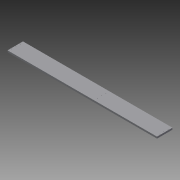
# Autodesk Inventor part: licht_200_back1
Saved by Autodesk Inventor 2015 (Build 190159000, 159)
## iProperties
Created: 2018-01-11
Part Number: licht_200_back1
Material: Generisch
Document SubType Name: Modeling
Designer: schueler
Density: 1 g/cm^3
Appearance: Vorgabe
Author: schueler
Autodesk Inventor part; units mm, degrees
ref_plane "YZ Plane" through (0, 0, 0) normal (1, 0, 0) x (0, 1, 0)
ref_plane "XZ Plane" through (0, 0, 0) normal (0, 1, 0) x (-1, 0, 0)
ref_plane "XY Plane" through (0, 0, 0) normal (0, 0, 1) x (1, 0, 0)
sketch "Skizze1" plane through (0, 0, 0) normal (0, 0, 1) x (1, 0, 0)
  line L0 (0, 0) -> (1392, 0)
  line L1 (1392, 0) -> (1392, 144)
  line L2 (1392, 144) -> (0, 144)
  line L3 (0, 144) -> (0, 0)
  line L4 (1384, 144) -> (1384, 0) construction
  line L5 (1392, 112) -> (0, 112) construction
  line L6 (1392, 32) -> (0, 32) construction
  circle A0 centre (1384, 112) radius 1.5
  circle A1 centre (1384, 32) radius 1.5
  line L7 (8, 144) -> (8, 0) construction
  circle A2 centre (8, 112) radius 1.5
  circle A3 centre (8, 72) radius 1.5
  circle A4 centre (8, 32) radius 1.5
  circle A5 centre (1384, 72) radius 1.5
  circle A6 centre (805, 112) radius 1.5
  circle A7 centre (805, 72) radius 1.5
  circle A8 centre (805, 32) radius 1.5
  line L8 (805, 144) -> (805, 0) construction
  point P0 (1392, 72)
  point P1 (805, 72)
  dimension "d0" = 1392
  dimension "d1" = 144
  dimension "d20" = 8
  dimension "d21" = 40
  dimension "d22" = 40
  dimension "d23" = 3
  dimension "d24" = 3
  dimension "d25" = 8
  dimension "d26" = 3
  dimension "d27" = 3
  dimension "d28" = 3
  dimension "d29" = 3
  dimension "d131" = 3
  dimension "d132" = 3
  dimension "d133" = 3
  dimension "d134" = 805
  constraints: 22 point on line, 18 end point, 9 centre point, 5 midpoint, 5 perpendicular, 3 parallel, 1 horizontal
  measures "d0" distance of L2.end L1.end
  measures "d1" distance of L1.end L0.end
  measures "d20" distance of L1.end L4.start
  measures "d21" distance of L5.start point (1392, 72)
  measures "d22" distance of L6.start point (1392, 72)
  measures "d23" diameter of A0
  measures "d24" diameter of A1
  measures "d25" distance of L7.start L2.end
  measures "d26" diameter of A2
  measures "d27" diameter of A3
  measures "d28" diameter of A4
  measures "d29" diameter of A5
  measures "d131" diameter of A6
  measures "d132" diameter of A7
  measures "d133" diameter of A8
  measures "d134" distance between parallel lines of L8 L3
extrude "Extrusion1" add sketch "Skizze1" along normal blind 16 contours L3 L2 L1 L0 | A6 | A7 | A8
sketch "Skizze2" plane through (0, 0, 16) normal (0, 0, 1) x (1, 0, 0)
  circle A0 centre (1384, 112) radius 1.5 projected
  circle A1 centre (1384, 72) radius 1.5 projected
  circle A2 centre (1384, 32) radius 1.5 projected
  circle A3 centre (8, 72) radius 1.5 projected
  circle A4 centre (8, 112) radius 1.5 projected
  circle A5 centre (8, 32) radius 1.5 projected
  circle A6 centre (805, 32) radius 1.5 projected
  circle A7 centre (805, 112) radius 1.5 projected
  circle A8 centre (805, 72) radius 1.5 projected
  point P0 (0, 0)
  point P1 (805, 72)
  point P2 (821.0338, 32)
  point P3 (821.0338, 72)
  constraints: 1 coincident
hole "Bohrung7" at (1384, 112, 16) at (1384, 72, 16) at (1384, 32, 16) at (8, 72, 16) at (8, 32, 16) at (8, 112, 16) at (805, 32, 16) at (805, 112, 16) at (805, 72, 16) at (805, 112, 16) at (805, 32, 16) at (805, 72, 16) at (805, 112, 16) direction (0, 0, -1) diameter 3 end through all countersink diameter 8 countersink angle 90
sketch "Skizze3" plane through (0, 144, 0) normal (0, 1, 0) x (1, 0, 0)
  line L0 (0, 0) -> (1392, 0) construction
  line L1 (1392, 0) -> (1392, -16) construction
  line L2 (1392, -16) -> (0, -16) construction
  line L3 (0, -16) -> (0, 0) construction
  line L4 (0, 0) -> (0, -16) projected
  line L5 (0, -8) -> (1392, -8) construction
  line L6 (1392, 0) -> (1392, -16) projected
  line L7 (0, -16) -> (1392, -16) construction
  line L8 (696, -16) -> (696, 0) construction
  point P0 (250, -8)
  point P1 (750, -8)
  point P2 (1250, -8)
  dimension "d135" = 500
  dimension "d136" = 500
  dimension "d137" = 250
  constraints: 12 end point, 4 midpoint, 3 point on line, 2 parallel, 1 horizontal, 1 perpendicular
  measures "d135" distance of point (750, -8) point (1250, -8)
  measures "d136" distance of point (250, -8) point (750, -8)
  measures "d137" distance from line of L4 point (250, -8)
hole "Bohrung12" at (250, 144, 8) at (750, 144, 8) at (1250, 144, 8) direction (0, -1, 0) diameter 3 depth 30 tip angle 118
